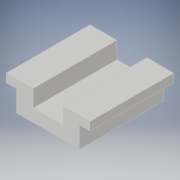
# Autodesk Inventor part: RS-FixedFiber
Saved by Autodesk Inventor 2019 (Build 230136000, 136)
## iProperties
Created: 2019-06-18
Part Number: RS-FixedFiber
Material: Generic
Document SubType Name: Modeling
Designer: aorfi
Density: 1 g/cm^3
Appearance: Default
Author: aorfi
Autodesk Inventor part; units mm, degrees
ref_plane "YZ Plane" through (0, 0, 0) normal (1, 0, 0) x (0, 1, 0)
ref_plane "XZ Plane" through (0, 0, 0) normal (0, 1, 0) x (-1, 0, 0)
ref_plane "XY Plane" through (0, 0, 0) normal (0, 0, 1) x (1, 0, 0)
sketch "Sketch1" plane through (0, 0, 0) normal (0, 1, 0) x (-1, 0, 0)
  line L0 (-10, 10) -> (10, 10)
  line L1 (10, 10) -> (10, -10)
  line L2 (10, -10) -> (-10, -10)
  line L3 (-10, -10) -> (-10, 10)
  line L4 (-10, 10) -> (10, -10) construction
  line L5 (10, 10) -> (-10, -10) construction
  point P0 (0, 0)
  dimension "d0" = 20
  dimension "d1" = 20
  constraints: 12 end point, 2 midpoint, 2 parallel, 1 horizontal, 1 perpendicular
  measures "d0" distance of L0.end L1.end
  measures "d1" distance of L1.end L2.end
extrude "Extrusion1" add sketch "Sketch1" along normal mid plane 3
sketch "Sketch2" plane through (0, 1.5, 0) normal (0, 1, 0) x (1, 0, 0)
  line L0 (-10, -10) -> (10, -10) projected
  line L1 (10, -10) -> (10, 10) projected
  line L2 (10, 10) -> (-10, 10) projected
  line L3 (-10, 10) -> (-10, -10) projected
  line L4 (-3.565, -10) -> (3.565, -10)
  line L5 (3.565, -10) -> (3.565, 10)
  line L6 (3.565, 10) -> (-3.565, 10)
  line L7 (-3.565, 10) -> (-3.565, -10)
  point P0 (0, 0)
  point P1 (0, 10)
  dimension "d5" = 7.13
  constraints: 8 end point, 2 parallel, 2 point on line, 1 horizontal, 1 midpoint, 1 perpendicular, 1 vertical alignment
  measures "d5" distance between parallel lines of L5 L7
extrude "Extrusion2" add sketch "Sketch2" along normal blind 4 contours L3 L2 L7 L0 | L5 L2 L1 L0
sketch "Sketch3" plane through (-10, -1.5, 10) normal (0, 0, 1) x (1, 0, 0)
  line L0 (0, 7) -> (0, 0) projected
  line L1 (2.5, 5) -> (0, 5)
  line L2 (0, 5) -> (0, 0)
  line L3 (0, 0) -> (2.5, 0)
  line L4 (2.5, 0) -> (2.5, 5)
  line L5 (2.5, 5) -> (0, 0) construction
  line L6 (0, 5) -> (2.5, 0) construction
  line L7 (20, 0) -> (0, 0) projected
  line L8 (17.5, 5) -> (20, 5)
  line L9 (20, 5) -> (20, 0)
  line L10 (20, 0) -> (17.5, 0)
  line L11 (17.5, 0) -> (17.5, 5)
  line L12 (17.5, 5) -> (20, 0) construction
  line L13 (20, 5) -> (17.5, 0) construction
  point P0 (10, 1.5)
  point P1 (1.25, 2.5)
  point P2 (18.75, 2.5)
  point P3 (1.25, 2.5)
  point P4 (18.75, 2.5)
  dimension "d8" = 2.5
  dimension "d9" = 5
  constraints: 24 end point, 6 midpoint, 4 parallel, 2 horizontal, 2 perpendicular, 1 collinear, 1 horizontal alignment
  measures "d8" distance of L1.start L1.end
  measures "d9" distance of L3.end L1.start
extrude "Extrusion3" cut sketch "Sketch3" against normal through all
body "Solid1"
